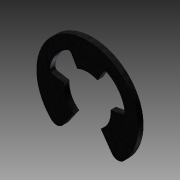
# Autodesk Inventor part: e-clip
Saved by Autodesk Inventor 2012 (Build 160160000, 160)
## iProperties
Created: 2009-01-30
Part Number: e-clip
Material: Steel, Mild
Document SubType Name: Modeling
Designer: Administrator
Density: 7.86 g/cm^3
Author: Administrator
Autodesk Inventor part; units mm, degrees
ref_plane "YZ Plane" through (0, 0, 0) normal (1, 0, 0) x (0, 1, 0)
ref_plane "XZ Plane" through (0, 0, 0) normal (0, 1, 0) x (-1, 0, 0)
ref_plane "XY Plane" through (0, 0, 0) normal (0, 0, 1) x (1, 0, 0)
sketch "Sketch1" plane through (0, 0, 0) normal (0, 0, 1) x (1, 0, 0)
  line L0 (-11.7348, 0) -> (11.7348, 0) projected
  line L1 (0, -9.2893) -> (0, 11.3272) projected
  arc A0 (5.9648, -5.8889) -> (-5.9648, -5.8889) centre (0, 0) ccw
  arc A1 (-5.9648, -5.8889) -> (-4.0207, -5.7251) centre (-5.061, -4.9966) ccw
  arc A2 (4.0207, -5.7251) -> (5.9648, -5.8889) centre (5.061, -4.9966) ccw
  line L2 (0, 0) -> (-6.8661, 4.8077) construction
  line L3 (0, 0) -> (6.8661, 4.8077) construction
  line L4 (4.0207, -5.7251) -> (2.2225, -3.1569)
  line L5 (-4.0207, -5.7251) -> (-2.2225, -3.1569)
  line L6 (1.6581, 3.4866) -> (2.642, 5.1906)
  line L7 (-1.6581, 3.4866) -> (-2.642, 5.1906)
  line L8 (-3.8434, 0.3656) -> (-5.7812, 0.7073)
  line L9 (3.8434, 0.3656) -> (5.7812, 0.7073)
  arc A3 (-3.274, 5.3751) -> (-6.1707, 1.2381) centre (-0.7559, 0.5293) ccw
  arc A4 (6.1707, 1.2381) -> (3.274, 5.3751) centre (0.7559, 0.5293) ccw
  arc A5 (-2.642, 5.1906) -> (-3.274, 5.3751) centre (-3.0544, 4.9525) ccw
  arc A6 (-6.1707, 1.2381) -> (-5.7812, 0.7073) centre (-5.6985, 1.1763) ccw
  arc A7 (3.274, 5.3751) -> (2.642, 5.1906) centre (3.0544, 4.9525) ccw
  arc A8 (5.7812, 0.7073) -> (6.1707, 1.2381) centre (5.6985, 1.1763) ccw
  arc A9 (-3.8434, 0.3656) -> (-2.2225, -3.1569) centre (0, 0) ccw
  arc A10 (2.2225, -3.1569) -> (3.8434, 0.3656) centre (0, 0) ccw
  arc A11 (1.6581, 3.4866) -> (-1.6581, 3.4866) centre (0, 0) ccw
  point P0 (2.8602, 5.5686)
  point P1 (-2.8602, 5.5686)
  point P2 (-6.211, 0.7831)
  point P3 (6.211, 0.7831)
  dimension "d19" = 1.27
  dimension "d30" = 8.382
  dimension "d35" = 35
  dimension "d36" = 35
  dimension "d37" = 4.445
  dimension "d38" = 30
  dimension "d39" = 2.4041
  dimension "d40" = 0.4763
  dimension "d41" = 3.8608
  dimension "d42" = 3.8608
  dimension "d43" = 3.8608
  dimension "d45" = 3.81
  dimension "d46" = 5.461
  constraints: 30 point on circle, 16 end point, 12 centre point, 12 tangent, 5 equal radius, 4 point on line, 3 equal length, 2 coincident, 2 perpendicular, 1 horizontal alignment, 3 other
  measures "d19" radius of A1
  measures "d30" radius of A0
  measures "d35" angle of L0 L3
  measures "d36" angle of L2 L0
  measures "d37" distance of L4.end L5.end
  measures "d38" angle of L1 L6
  measures "d39" distance of L8.start point (-6.211, 0.783)
  measures "d40" radius of A5
  measures "d41" radius of A10
  measures "d42" radius of A9
  measures "d43" radius of A11
  measures "d45" distance of L7.start L8.start
  measures "d46" radius of A3
extrude "Extrusion2" add sketch "Sketch1" along normal mid plane 0.889 contours A0 L1 A11 L7 A5 A3 A6 L8 A9 L0 | L0 A9 L5 A1 A0 | A0 L0 A10 L9 A8 A4 A7 L6 A11 L1 | A0 A2 L4 A10 L0
body "Solid2"
